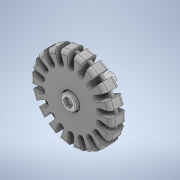
# Autodesk Inventor part: wheel_simplified2
Saved by Autodesk Inventor 2021 (Build 250183000, 183)
## iProperties
Created: 2022-09-21
Part Number: wheel_simplified2
Material: Generic
Document SubType Name: Modeling
Designer: victo
Density: 1 g/cm^3
Appearance: Default
Author: victo
Autodesk Inventor part; units mm, degrees
ref_plane "YZ Plane" through (0, 0, 0) normal (1, 0, 0) x (0, 1, 0)
ref_plane "XZ Plane" through (0, 0, 0) normal (0, 1, 0) x (-1, 0, 0)
ref_plane "XY Plane" through (0, 0, 0) normal (0, 0, 1) x (1, 0, 0)
sketch "Sketch1" plane through (0, 0, 0) normal (0, 0, 1) x (1, 0, 0)
  circle A0 centre (0, 0) radius 22.5
  circle A1 centre (0, 0) radius 5
  line L0 (0, 22.95) -> (0, 16.25) construction
  line L1 (-1.6, 22.95) -> (-1.6, 16.25)
  line L2 (1.6, 16.25) -> (1.6, 22.95)
  arc A2 (1.6, 22.95) -> (-1.6, 22.95) centre (0, 22.95) ccw
  arc A3 (-1.6, 16.25) -> (1.6, 16.25) centre (0, 16.25) ccw
  line L3 (-9.3529, 21.0187) -> (-7.0613, 14.7228)
  arc A4 (-6.3459, 22.1132) -> (-9.3529, 21.0187) centre (-7.8494, 21.5659) ccw
  line L4 (-7.8494, 21.5659) -> (-5.5578, 15.27) construction
  line L5 (-4.0543, 15.8172) -> (-6.3459, 22.1132)
  arc A5 (-7.0613, 14.7228) -> (-4.0543, 15.8172) centre (-5.5578, 15.27) ccw
  line L6 (-15.9776, 16.5523) -> (-11.671, 11.4198)
  arc A6 (-13.5263, 18.6092) -> (-15.9776, 16.5523) centre (-14.752, 17.5807) ccw
  line L7 (-14.752, 17.5807) -> (-10.4453, 12.4482) construction
  line L8 (-9.2196, 13.4767) -> (-13.5263, 18.6092)
  arc A7 (-11.671, 11.4198) -> (-9.2196, 13.4767) centre (-10.4453, 12.4482) ccw
  line L9 (-20.6753, 10.0894) -> (-14.8729, 6.7394)
  arc A8 (-19.0753, 12.8606) -> (-20.6753, 10.0894) centre (-19.8753, 11.475) ccw
  line L10 (-19.8753, 11.475) -> (-14.0729, 8.125) construction
  line L11 (-13.2729, 9.5106) -> (-19.0753, 12.8606)
  arc A9 (-14.8729, 6.7394) -> (-13.2729, 9.5106) centre (-14.0729, 8.125) ccw
  line L12 (-22.8792, 2.4095) -> (-16.281, 1.2461)
  arc A10 (-22.3235, 5.5609) -> (-22.8792, 2.4095) centre (-22.6013, 3.9852) ccw
  line L13 (-22.6013, 3.9852) -> (-16.0031, 2.8218) construction
  line L14 (-15.7253, 4.3975) -> (-22.3235, 5.5609)
  arc A11 (-16.281, 1.2461) -> (-15.7253, 4.3975) centre (-16.0031, 2.8218) ccw
  line L15 (-22.3235, -5.5609) -> (-15.7253, -4.3975)
  arc A12 (-22.8792, -2.4095) -> (-22.3235, -5.5609) centre (-22.6013, -3.9852) ccw
  line L16 (-22.6013, -3.9852) -> (-16.0031, -2.8218) construction
  line L17 (-16.281, -1.2461) -> (-22.8792, -2.4095)
  arc A13 (-15.7253, -4.3975) -> (-16.281, -1.2461) centre (-16.0031, -2.8218) ccw
  line L18 (-19.0753, -12.8606) -> (-13.2729, -9.5106)
  arc A14 (-20.6753, -10.0894) -> (-19.0753, -12.8606) centre (-19.8753, -11.475) ccw
  line L19 (-19.8753, -11.475) -> (-14.0729, -8.125) construction
  line L20 (-14.8729, -6.7394) -> (-20.6753, -10.0894)
  arc A15 (-13.2729, -9.5106) -> (-14.8729, -6.7394) centre (-14.0729, -8.125) ccw
  line L21 (-13.5263, -18.6092) -> (-9.2196, -13.4767)
  arc A16 (-15.9776, -16.5523) -> (-13.5263, -18.6092) centre (-14.752, -17.5807) ccw
  line L22 (-14.752, -17.5807) -> (-10.4453, -12.4482) construction
  line L23 (-11.671, -11.4198) -> (-15.9776, -16.5523)
  arc A17 (-9.2196, -13.4767) -> (-11.671, -11.4198) centre (-10.4453, -12.4482) ccw
  line L24 (-6.3459, -22.1132) -> (-4.0543, -15.8172)
  arc A18 (-9.3529, -21.0187) -> (-6.3459, -22.1132) centre (-7.8494, -21.5659) ccw
  line L25 (-7.8494, -21.5659) -> (-5.5578, -15.27) construction
  line L26 (-7.0613, -14.7228) -> (-9.3529, -21.0187)
  arc A19 (-4.0543, -15.8172) -> (-7.0613, -14.7228) centre (-5.5578, -15.27) ccw
  line L27 (1.6, -22.95) -> (1.6, -16.25)
  arc A20 (-1.6, -22.95) -> (1.6, -22.95) centre (0, -22.95) ccw
  line L28 (0, -22.95) -> (0, -16.25) construction
  line L29 (-1.6, -16.25) -> (-1.6, -22.95)
  arc A21 (1.6, -16.25) -> (-1.6, -16.25) centre (0, -16.25) ccw
  line L30 (9.3529, -21.0187) -> (7.0613, -14.7228)
  arc A22 (6.3459, -22.1132) -> (9.3529, -21.0187) centre (7.8494, -21.5659) ccw
  line L31 (7.8494, -21.5659) -> (5.5578, -15.27) construction
  line L32 (4.0543, -15.8172) -> (6.3459, -22.1132)
  arc A23 (7.0613, -14.7228) -> (4.0543, -15.8172) centre (5.5578, -15.27) ccw
  line L33 (15.9776, -16.5523) -> (11.671, -11.4198)
  arc A24 (13.5263, -18.6092) -> (15.9776, -16.5523) centre (14.752, -17.5807) ccw
  line L34 (14.752, -17.5807) -> (10.4453, -12.4482) construction
  line L35 (9.2196, -13.4767) -> (13.5263, -18.6092)
  arc A25 (11.671, -11.4198) -> (9.2196, -13.4767) centre (10.4453, -12.4482) ccw
  line L36 (20.6753, -10.0894) -> (14.8729, -6.7394)
  arc A26 (19.0753, -12.8606) -> (20.6753, -10.0894) centre (19.8753, -11.475) ccw
  line L37 (19.8753, -11.475) -> (14.0729, -8.125) construction
  line L38 (13.2729, -9.5106) -> (19.0753, -12.8606)
  arc A27 (14.8729, -6.7394) -> (13.2729, -9.5106) centre (14.0729, -8.125) ccw
  line L39 (22.8792, -2.4095) -> (16.281, -1.2461)
  arc A28 (22.3235, -5.5609) -> (22.8792, -2.4095) centre (22.6013, -3.9852) ccw
  line L40 (22.6013, -3.9852) -> (16.0031, -2.8218) construction
  line L41 (15.7253, -4.3975) -> (22.3235, -5.5609)
  arc A29 (16.281, -1.2461) -> (15.7253, -4.3975) centre (16.0031, -2.8218) ccw
  line L42 (22.3235, 5.5609) -> (15.7253, 4.3975)
  arc A30 (22.8792, 2.4095) -> (22.3235, 5.5609) centre (22.6013, 3.9852) ccw
  line L43 (22.6013, 3.9852) -> (16.0031, 2.8218) construction
  line L44 (16.281, 1.2461) -> (22.8792, 2.4095)
  arc A31 (15.7253, 4.3975) -> (16.281, 1.2461) centre (16.0031, 2.8218) ccw
  line L45 (19.0753, 12.8606) -> (13.2729, 9.5106)
  arc A32 (20.6753, 10.0894) -> (19.0753, 12.8606) centre (19.8753, 11.475) ccw
  line L46 (19.8753, 11.475) -> (14.0729, 8.125) construction
  line L47 (14.8729, 6.7394) -> (20.6753, 10.0894)
  arc A33 (13.2729, 9.5106) -> (14.8729, 6.7394) centre (14.0729, 8.125) ccw
  line L48 (13.5263, 18.6092) -> (9.2196, 13.4767)
  arc A34 (15.9776, 16.5523) -> (13.5263, 18.6092) centre (14.752, 17.5807) ccw
  line L49 (14.752, 17.5807) -> (10.4453, 12.4482) construction
  line L50 (11.671, 11.4198) -> (15.9776, 16.5523)
  arc A35 (9.2196, 13.4767) -> (11.671, 11.4198) centre (10.4453, 12.4482) ccw
  line L51 (6.3459, 22.1132) -> (4.0543, 15.8172)
  arc A36 (9.3529, 21.0187) -> (6.3459, 22.1132) centre (7.8494, 21.5659) ccw
  line L52 (7.8494, 21.5659) -> (5.5578, 15.27) construction
  line L53 (7.0613, 14.7228) -> (9.3529, 21.0187)
  arc A37 (4.0543, 15.8172) -> (7.0613, 14.7228) centre (5.5578, 15.27) ccw
  point P0 (0, 19.6)
  point P1 (-1.6, 22.443)
  point P2 (-6.1725, 21.6368)
  point P3 (-9.1795, 20.5423)
  point P4 (-13.2004, 18.2208)
  point P5 (-15.6518, 16.1639)
  point P6 (-18.6362, 12.6072)
  point P7 (-20.2362, 9.8359)
  point P8 (-21.8242, 5.4729)
  point P9 (-22.3799, 2.3215)
  point P10 (-22.3799, -2.3215)
  point P11 (-21.8242, -5.4729)
  point P12 (-20.2362, -9.8359)
  point P13 (-18.6362, -12.6072)
  point P14 (-15.6518, -16.1639)
  point P15 (-13.2004, -18.2208)
  point P16 (-9.1795, -20.5423)
  point P17 (-6.1725, -21.6368)
  point P18 (-1.6, -22.443)
  point P19 (1.6, -22.443)
  point P20 (6.1725, -21.6368)
  point P21 (9.1795, -20.5423)
  point P22 (13.2004, -18.2208)
  point P23 (15.6518, -16.1639)
  point P24 (18.6362, -12.6072)
  point P25 (20.2362, -9.8359)
  point P26 (21.8242, -5.4729)
  point P27 (22.3799, -2.3215)
  point P28 (22.3799, 2.3215)
  point P29 (21.8242, 5.4729)
  point P30 (20.2362, 9.8359)
  point P31 (18.6362, 12.6072)
  point P32 (15.6518, 16.1639)
  point P33 (13.2004, 18.2208)
  point P34 (9.1795, 20.5423)
  point P35 (6.1725, 21.6368)
  point P36 (1.6, 22.443)
  dimension "d0" = 45
  dimension "d1" = 10
  dimension "d2" = 3.2
  dimension "d3" = 3.35
  dimension "d4" = 19.6
  dimension "d5" = 0
  dimension "d8" = 360
  constraints: 144 end point, 72 point on circle, 37 centre point, 4 tangent, 2 coincident, 1 midpoint, 1 parallel, 1 vertical, 201 other
  measures "d1" diameter of A1
  measures "d2" diameter of A3
  measures "d3" distance of L0.end point (0, 19.6)
  measures "d4" distance of point (0, 0) point (0, 19.6)
  measures "d5" horizontal distance of point (0, 0) point (0, 19.6)
extrude "Extrusion1" add sketch "Sketch1" along normal blind 8.5 contours A0 L39 A29 L41 L36 A27 L38 L33 A25 L35 L30 A23 L32 L27 A21 L29 L24 A19 L26 L21 A17 L23 L18 A15 L20 L15 A13 L17 L12 A11 L14 L9 A9 L11 L6 A7 L8 L3 A5 L5 L1 A3 L2 L51 A37 L53 L48 A35 L50 L45 A33 L47 L42 A31 L44
sketch "Sketch2" plane through (0, 0, 0) normal (0, 0, -1) x (-1, 0, 0)
  circle A0 centre (0, 0) radius 13.5
  circle A1 centre (0, 0) radius 5 projected
  dimension "d12" = 27
  constraints: 1 centre point, 1 coincident
  measures "d12" diameter of A0
extrude "Extrusion2" add sketch "Sketch2" along normal blind 2
sketch "Sketch3" plane through (0, 0, 0) normal (1, 0, 0) x (0, 1, 0)
  line L0 (-16.25, 0) -> (-22.443, 0) projected
  line L1 (-22.443, 0) -> (-22.443, 8.5) projected
  line L2 (-16.25, 8.5) -> (-22.443, 8.5) projected
  line L3 (-16.25, 0) -> (-16.25, 8.5) projected
  line L4 (-22.443, 3.9) -> (-16.1639, 3.9) construction
  line L5 (-16.1639, 0) -> (-16.1639, 8.5) projected
  circle A0 centre (-20.343, 3.9) radius 0.95
  point P0 (0, 0)
  dimension "d15" = 4.6
  dimension "d16" = 1.9
  dimension "d17" = 2.1
  constraints: 3 point on line, 2 end point, 1 centre point, 1 horizontal
  measures "d15" distance between parallel lines of L2 L4
  measures "d16" diameter of A0
  measures "d17" distance from line of L1 A0.centre
extrude "Extrusion3" add sketch "Sketch3" against normal mid plane 3.2 contours A0
pattern_circular "Circular Pattern1" count 18 over 360 about axis through (0, 0, 0) along (0, 0, 1) of "Extrusion3"
sketch "Sketch4" plane through (0, 0, 8.5) normal (0, 0, 1) x (1, 0, 0)
  circle A0 centre (0, 0) radius 5 projected
  circle A1 centre (0, 0) radius 4.25
  dimension "d23" = 8.5
  constraints: 1 centre point, 1 coincident
  measures "d23" diameter of A1
extrude "Extrusion4" add sketch "Sketch4" along normal blind 1.5 and the other way blind 1.7 contours A1
sketch "Sketch5" plane through (0, 0, 10) normal (0, 0, 1) x (1, 0, 0)
  circle A0 centre (0, 0) radius 4.25 projected
  line L0 (1.3279, 2.3) -> (2.6558, 0)
  line L1 (2.6558, 0) -> (1.3279, -2.3)
  line L2 (1.3279, -2.3) -> (-1.3279, -2.3)
  line L3 (-1.3279, -2.3) -> (-2.6558, 0)
  line L4 (-2.6558, 0) -> (-1.3279, 2.3)
  line L5 (-1.3279, 2.3) -> (1.3279, 2.3)
  dimension "d28" = 4.6
  constraints: 12 end point, 1 coincident, 1 horizontal, 13 other
  measures "d28" distance between parallel lines of L2 L5
extrude "Extrusion5" cut sketch "Sketch5" against normal blind 2 contours L0 L1 L2 L3 L4 L5
sketch "Sketch6" plane through (0, 0, 6.8) normal (0, 0, -1) x (-1, 0, 0)
  circle A0 centre (0, 0) radius 5 projected
extrude "Extrusion6" add sketch "Sketch6" along normal blind 21
sketch "Sketch7" plane through (0, 0, -14.2) normal (0, 0, -1) x (-1, 0, 0)
  circle A0 centre (0, 0) radius 5 projected
  circle A1 centre (0, 0) radius 2.5
  dimension "d33" = 5
  constraints: 1 centre point, 1 coincident
  measures "d33" diameter of A1
extrude "Extrusion7" cut sketch "Sketch7" against normal up to surface (12.2 mm away)
fillet "Fillet1" radius 2 36 edges at (11.25, -19.4856, 8.5) (11.25, -19.4856, 0) (3.9071, -22.1582, 8.5) (3.9071, -22.1582, 0) (-3.9071, -22.1582, 8.5) (-3.9071, -22.1582, 0) (-11.25, -19.4856, 8.5) (-11.25, -19.4856, 0) (-17.236, -14.4627, 8.5) (-17.236, -14.4627, 0) (-21.1431, -7.6955, 8.5) (-21.1431, -7.6955, 0) (-22.5, 0, 8.5) (-22.5, 0, 0) (-21.1431, 7.6955, 8.5) (-21.1431, 7.6955, 0) (-17.236, 14.4627, 8.5) (-17.236, 14.4627, 0) (-11.25, 19.4856, 8.5) (-11.25, 19.4856, 0) (-3.9071, 22.1582, 8.5) (-3.9071, 22.1582, 0) (3.9071, 22.1582, 8.5) (3.9071, 22.1582, 0) (11.25, 19.4856, 8.5) (11.25, 19.4856, 0) (17.236, 14.4627, 8.5) (17.236, 14.4627, 0) (21.1431, 7.6955, 8.5) (21.1431, 7.6955, 0) (22.5, 0, 8.5) (22.5, 0, 0) (21.1431, -7.6955, 8.5) (21.1431, -7.6955, 0) (17.236, -14.4627, 8.5) (17.236, -14.4627, 0)
fillet "Fillet1" radius 0.5 1 edges at (-4.25, 0, 10)
body "Solid1"
